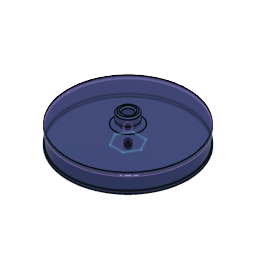
FEKTBOT_wheel_shaft_ver_1_2 (Autodesk Fusion 360 design; units mm, degrees)
Autodesk Fusion 360 part; units mm, degrees
sketch "spodek" plane through (0, 0, 0) normal (0, 1, 0) x (1, 0, 0)
  circle A0 centre (0, 0) radius 31.75
  circle A1 centre (0, 0) radius 1
  dimension "d1" = 63.5
  dimension "d2" = 2
  constraint coincident A0.centre A1.centre
  measures "d1" diameter of A0
  measures "d2" diameter of A1
extrude "Extrude1" add sketch "spodek" along normal blind 1.5
sketch "prostredek" plane through (0, 1.5, 0) normal (0, 1, 0) x (-1, 0, 0)
  circle A0 centre (0, 0) radius 1
  circle A1 centre (0, 0) radius 31.75
  circle A2 centre (0, 0) radius 31.55
  line L0 (3.493, -6.05) -> (6.9859, 0)
  line L1 (6.9859, 0) -> (3.493, 6.05)
  line L2 (3.493, 6.05) -> (-3.493, 6.05)
  line L3 (-3.493, 6.05) -> (-6.9859, 0)
  line L4 (-6.9859, 0) -> (-3.493, -6.05)
  line L5 (-3.493, -6.05) -> (3.493, -6.05)
  dimension "d5" = -0.2
  dimension "d6" = 6.05
  constraint coincident A0.centre A1.centre
  measures "d6" distance of A0.centre L5
extrude "Extrude2" add sketch "prostredek" along normal blind 7 contours A2 | L0 L1 L2 L3 L4 L5
sketch "Sketch3" plane through (0, 8.5, 0) normal (0, 1, 0) x (-1, 0, 0)
  circle A0 centre (0, 0) radius 31.75
  line L0 (-1.4902, 2.1) -> (1.4902, 2.1)
  arc A1 (-1.4902, 2.1) -> (1.4902, 2.1) centre (0, 0) ccw
  dimension "d12" = 5.15
  dimension "d13" = 2.1
  constraint concentric A0 A1
  constraint horizontal L0
  measures "d12" diameter of A1
  measures "d13" distance of A0.centre L0
extrude "Extrude4" cut sketch "Sketch3" against normal blind 6 contours L0 A1
extrude "Extrude5" add sketch "Sketch3" along normal blind 1.5
sketch "Sketch4" plane through (0, 10, 0) normal (0, 1, 0) x (-1, 0, 0)
  arc A0 (-1.4902, 2.1) -> (1.4902, 2.1) centre (0, 0) ccw
  line L0 (-1.4902, 2.1) -> (1.4902, 2.1)
  circle A1 centre (0, 0) radius 31.75
  circle A2 centre (0, 0) radius 5
  dimension "d22" = 10
  constraint coincident A0.centre A1.centre
  measures "d22" diameter of A2
extrude "Extrude6" add sketch "Sketch4" along normal blind 6 contours A2
fillet "Fillet3" radius 0.8 1 faces at (-0.1246, 16, 3.062)
fillet "Fillet4" radius 2 1 edges at (4.6616, 10, 1.8081)
